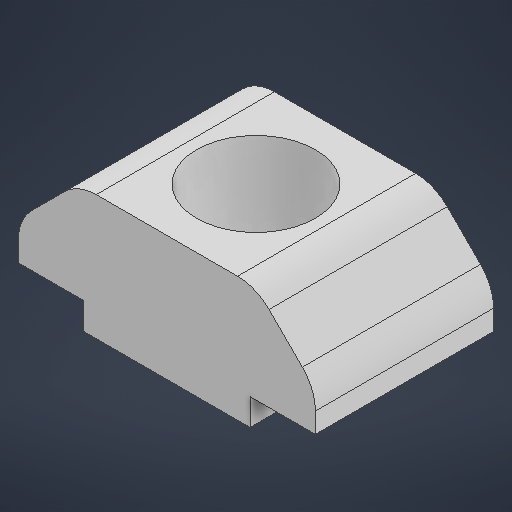
# Autodesk Inventor part: M4 T-Slot Nut
Saved by Autodesk Inventor 2025.1 (Build 291241000, 241)
## iProperties
Created: 2025-01-21
Part Number: M4 T-Slot Nut
Material: Generic
Document SubType Name: Modeling
Designer: jerem
Density: 1 g/cm^3
Appearance: Default
Author: jerem
Autodesk Inventor part; units mm, degrees
ref_plane "YZ Plane" through (0, 0, 0) normal (1, 0, 0) x (0, 1, 0)
ref_plane "XZ Plane" through (0, 0, 0) normal (0, 1, 0) x (-1, 0, 0)
ref_plane "XY Plane" through (0, 0, 0) normal (0, 0, 1) x (1, 0, 0)
sketch "Sketch1" plane through (0, 0, 0) normal (0, 1, 0) x (-1, 0, 0)
  line L0 (-5, -3) -> (5, -3)
  line L1 (5, -3) -> (5, 3)
  line L2 (5, 3) -> (-5, 3)
  line L3 (-5, 3) -> (-5, -3)
  line L4 (-5, -3) -> (5, 3) construction
  line L5 (5, -3) -> (-5, 3) construction
  line L6 (2.8, 3) -> (2.8, -3)
  line L7 (-2.8, -3) -> (-2.8, 3)
  line L8 (-2.8, 0) -> (2.8, 0) construction
  circle A0 centre (0, 0) radius 2
  dimension "d0" = 10
  dimension "d1" = 6
  dimension "d5" = 5.6
  dimension "d11" = 4
  constraints: 18 end point, 5 midpoint, 4 perpendicular, 4 point on line, 2 parallel, 1 centre point, 1 coincident, 1 horizontal
  measures "d0" distance of L2.end L1.end
  measures "d1" distance of L1.end L0.end
  measures "d5" distance between parallel lines of L7 L6
  measures "d11" diameter of A0
extrude "Extrusion1" add sketch "Sketch1" along normal blind 4.2
extrude "Extrusion2" cut sketch "Sketch1" along normal blind 0.9 contours L3 L2 L7 L0 | L6 L2 L1 L0
chamfer "Chamfer1" distance 2 angle 45 2 edges at (-5, 4.2, 0) (5, 4.2, 0)
fillet "Fillet1" radius 1.5 4 edges at (-3, 4.2, 0) (3, 4.2, 0) (-5, 2.2, 0) (5, 2.2, 0)
body "Solid1"
